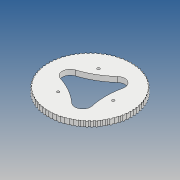
# Autodesk Inventor part: Plato Correa 2
Saved by Autodesk Inventor 2017 (Build 210142000, 142)
## iProperties
Part Number: Plato Correa 2
Material: Genérico
Document SubType Name: Modeling
Designer: FABLAB
Density: 1 g/cm^3
Appearance: Blanco
Author: FABLAB
Autodesk Inventor part; units mm, degrees
ref_plane "YZ Plane" through (0, 0, 0) normal (1, 0, 0) x (0, 1, 0)
ref_plane "XZ Plane" through (0, 0, 0) normal (0, 1, 0) x (-1, 0, 0)
ref_plane "XY Plane" through (0, 0, 0) normal (0, 0, 1) x (1, 0, 0)
sketch "Boceto1" plane through (0, 0, 0) normal (0, 0, 1) x (1, 0, 0)
  circle A0 centre (26.75, 0) radius 1.5 projected
  arc A1 (20.168, 17.783) -> (20.168, -17.783) centre (101.6471, 0) ccw projected
  arc A2 (5.3165, -26.3575) -> (20.168, -17.783) centre (11.375, -19.7021) ccw projected
  arc A3 (5.3165, -26.3575) -> (-25.4845, -8.5745) centre (-50.8235, -88.0289) ccw projected
  arc A4 (-25.4845, 8.5745) -> (-25.4845, -8.5745) centre (-22.75, 0) ccw projected
  arc A5 (-25.4845, 8.5745) -> (5.3165, 26.3575) centre (-50.8235, 88.0289) ccw projected
  arc A6 (20.168, 17.783) -> (5.3165, 26.3575) centre (11.375, 19.7021) ccw projected
  arc A7 (44.7856, -20.7385) -> (-44.7856, -20.7385) centre (0, 0) ccw construction
  circle A8 centre (-13.375, 23.1662) radius 1.5 projected
  circle A9 centre (-13.375, -23.1662) radius 1.5 projected
  circle A10 centre (47.3542, 0) radius 1
  line L0 (0, 0) -> (0, -72) construction
  arc A11 (-17.332, -80.0258) -> (17.332, -80.0258) centre (0, -72) ccw construction
  line L1 (17.332, -80.0258) -> (44.7856, -20.7385) construction
  line L2 (-17.332, -80.0258) -> (-44.7856, -20.7385) construction
  circle A12 centre (47.1882, 3.9625) radius 1
  circle A13 centre (46.6911, 7.8972) radius 1
  circle A14 centre (45.8665, 11.7765) radius 1
  circle A15 centre (44.7202, 15.5732) radius 1
  circle A16 centre (43.2602, 19.2607) radius 1
  circle A17 centre (41.4968, 22.8131) radius 1
  circle A18 centre (39.4423, 26.2054) radius 1
  circle A19 centre (37.1112, 29.414) radius 1
  circle A20 centre (34.5197, 32.4162) radius 1
  circle A21 centre (31.6862, 35.1911) radius 1
  circle A22 centre (28.6303, 37.7191) radius 1
  circle A23 centre (25.3737, 39.9825) radius 1
  circle A24 centre (21.939, 41.9655) radius 1
  circle A25 centre (18.3505, 43.6541) radius 1
  circle A26 centre (14.6333, 45.0365) radius 1
  circle A27 centre (10.8134, 46.1031) radius 1
  circle A28 centre (6.9176, 46.8462) radius 1
  circle A29 centre (2.9734, 47.2608) radius 1
  circle A30 centre (-0.9917, 47.3438) radius 1
  circle A31 centre (-4.9499, 47.0948) radius 1
  circle A32 centre (-8.8733, 46.5155) radius 1
  circle A33 centre (-12.7345, 45.6098) radius 1
  circle A34 centre (-16.5064, 44.3843) radius 1
  circle A35 centre (-20.1625, 42.8474) radius 1
  circle A36 centre (-23.6771, 41.01) radius 1
  circle A37 centre (-27.0257, 38.8849) radius 1
  circle A38 centre (-30.1847, 36.4871) radius 1
  circle A39 centre (-33.132, 33.8333) radius 1
  circle A40 centre (-35.8469, 30.9422) radius 1
  circle A41 centre (-38.3104, 27.8341) radius 1
  circle A42 centre (-40.5051, 24.5308) radius 1
  circle A43 centre (-42.4157, 21.0554) radius 1
  circle A44 centre (-44.0288, 17.4323) radius 1
  circle A45 centre (-45.3331, 13.6869) radius 1
  circle A46 centre (-46.3194, 9.8455) radius 1
  circle A47 centre (-46.9808, 5.9351) radius 1
  circle A48 centre (-47.3127, 1.983) radius 1
  circle A49 centre (-47.3127, -1.983) radius 1
  circle A50 centre (-46.9808, -5.9351) radius 1
  circle A51 centre (-46.3194, -9.8455) radius 1
  circle A52 centre (-45.3331, -13.6869) radius 1
  circle A53 centre (-44.0288, -17.4323) radius 1
  circle A54 centre (-42.4157, -21.0554) radius 1
  circle A55 centre (-40.5051, -24.5308) radius 1
  circle A56 centre (-38.3104, -27.8341) radius 1
  circle A57 centre (-35.8469, -30.9422) radius 1
  circle A58 centre (-33.132, -33.8333) radius 1
  circle A59 centre (-30.1847, -36.4871) radius 1
  circle A60 centre (-27.0257, -38.8849) radius 1
  circle A61 centre (-23.6771, -41.01) radius 1
  circle A62 centre (-20.1625, -42.8474) radius 1
  circle A63 centre (-16.5064, -44.3843) radius 1
  circle A64 centre (-12.7345, -45.6098) radius 1
  circle A65 centre (-8.8733, -46.5155) radius 1
  circle A66 centre (-4.9499, -47.0948) radius 1
  circle A67 centre (-0.9917, -47.3438) radius 1
  circle A68 centre (2.9734, -47.2608) radius 1
  circle A69 centre (6.9176, -46.8462) radius 1
  circle A70 centre (10.8134, -46.1031) radius 1
  circle A71 centre (14.6333, -45.0365) radius 1
  circle A72 centre (18.3505, -43.6541) radius 1
  circle A73 centre (21.939, -41.9655) radius 1
  arc A74 (-44.7856, -20.7385) -> (44.7856, -20.7385) centre (0, 0) ccw construction
  circle A75 centre (25.3737, -39.9825) radius 1
  circle A76 centre (0, 0) radius 47.3542
  circle A77 centre (0, 0) radius 46.3542 construction
  circle A78 centre (28.6303, -37.7191) radius 1
  circle A79 centre (31.6862, -35.1911) radius 1
  circle A80 centre (34.5197, -32.4162) radius 1
  circle A81 centre (37.1112, -29.414) radius 1
  circle A82 centre (39.4423, -26.2054) radius 1
  circle A83 centre (41.4968, -22.8131) radius 1
  circle A84 centre (43.2602, -19.2607) radius 1
  circle A85 centre (44.7202, -15.5732) radius 1
  arc A86 (17.332, -80.0258) -> (-17.332, -80.0258) centre (0, -72) ccw construction
  circle A87 centre (45.8665, -11.7765) radius 1
  circle A88 centre (46.6911, -7.8972) radius 1
  circle A89 centre (47.1882, -3.9625) radius 1
  dimension "d0" = 98.7085
  dimension "d9" = 2
  dimension "d11" = 72
  dimension "d20" = 43.4385
  dimension "d21" = 197.8912
  dimension "d22" = 65.3351
  dimension "radio" = 19.1
  dimension "d26" = 360
  dimension "d28" = 3.966
  dimension "d31" = 3
  dimension "d32" = 2
  constraints: 80 centre point, 8 point on circle, 8 tangent, 6 end point, 4 coincident, 2 horizontal alignment, 1 vertical, 153 other
  measures "d0" diameter of A7
  measures "d9" diameter of A10
  measures "d11" distance of L0.start L0.end
  measures "d22" distance of L1.start L1.end
  measures "radio" radius of A11
  measures "d28" distance of A18.centre A19.centre
  measures "d31" radial gap between concentric circles of A77 A7
extrude "Extrusión1" add sketch "Boceto1" along normal blind 6
sketch "Boceto2" plane through (0, 0, 6) normal (0, 0, 1) x (1, 0, 0)
  circle A0 centre (0, 0) radius 41.5
  arc A1 (20.168, 17.783) -> (20.168, -17.783) centre (101.6471, 0) ccw
  arc A2 (20.168, 17.783) -> (5.3165, 26.3575) centre (11.375, 19.7021) ccw projected
  arc A3 (-25.4845, 8.5745) -> (5.3165, 26.3575) centre (-50.8235, 88.0289) ccw
  arc A4 (-25.4845, 8.5745) -> (-25.4845, -8.5745) centre (-22.75, 0) ccw
  arc A5 (5.3165, -26.3575) -> (-25.4845, -8.5745) centre (-50.8235, -88.0289) ccw projected
  arc A6 (5.3165, -26.3575) -> (20.168, -17.783) centre (11.375, -19.7021) ccw projected
  circle A7 centre (-13.375, -23.1662) radius 1.5 projected
  circle A8 centre (-13.375, 23.1662) radius 1.5 projected
  circle A9 centre (26.75, 0) radius 1.5 projected
  dimension "d30" = 83
  constraints: 6 point on circle, 4 centre point, 1 coincident, 11 other
  measures "d30" diameter of A0
sketch "Boceto3" plane through (0, 0, 0) normal (0, 0, -1) x (-1, 0, 0)
  circle A0 centre (0, 0) radius 41.5 projected
  circle A1 centre (0, 0) radius 36
  point P0 (0, 0)
  dimension "d6" = 5.5
  constraints: 1 centre point
  measures "d6" radial gap between concentric circles of A0 A1
